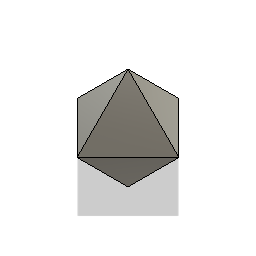
Octahedron_v1 (Autodesk Fusion 360 design; units mm, degrees)
Autodesk Fusion 360 part; units mm, degrees
sketch "Sketch1" plane through (0, 0, 0) normal (0, 1, 0) x (1, 0, 0)
  line L0 (0, 20) -> (20, 0)
  line L1 (20, 0) -> (0, -20)
  line L2 (0, -20) -> (-20, 0)
  line L3 (-20, 0) -> (0, 20)
  line L4 (0, -20) -> (0, 20) construction
  dimension "d1" = 40
sketch "Sketch2" plane through (0, 0, 0) normal (0, 0, 1) x (1, 0, 0)
  line L0 (0, 20) -> (0, -20)
  dimension "d2" = 40
loft "Loft1" add profiles "Sketch1" section 1 section 2 point at (0, -20, 0)
loft "Loft2" add section 1 face at (-6.6667, 0, 0) section 2 point at (0, 20, 0)
